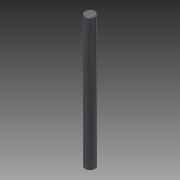
# Autodesk Inventor part: linear-guide-z
Saved by Autodesk Inventor 2012 SP1 (Build 160190100, 190)
## iProperties
Company: Taomaker.com
Created: 2011-11-06
Part Number: linear-guide-z
Material: Galvanized Steel
Document SubType Name: Modeling
Designer: Aaron Zhang
Mass: 80.0903 g
Surface Area: 42.221 cm^2
Volume: 10.2026 cm^3
Density: 7.85 g/cm^3
Title: Linear-Guide-Z-130mm
Author: Aaron Zhang
Autodesk Inventor part; units mm, degrees
ref_plane "YZ Plane" through (0, 0, 0) normal (1, 0, 0) x (0, 1, 0)
ref_plane "XZ Plane" through (0, 0, 0) normal (0, 1, 0) x (-1, 0, 0)
ref_plane "XY Plane" through (0, 0, 0) normal (0, 0, 1) x (1, 0, 0)
sketch "Sketch1" plane through (0, 0, 0) normal (0, 0, 1) x (1, 0, 0)
  circle A0 centre (0, 0) radius 5
  dimension "d0" = 10
  constraints: 1 centre point, 1 coincident
  measures "d0" diameter of A0
extrude "Extrusion1" add sketch "Sketch1" along normal blind 130
chamfer "Chamfer1" distance 0.5 angle 45 2 edges at (-5, 0, 130) (-5, 0, 0)
body "Solid1"
